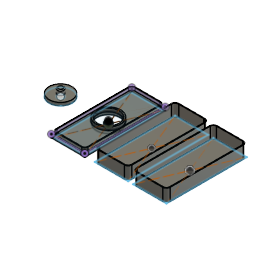
insert (Autodesk Fusion 360 design; units mm, degrees)
Autodesk Fusion 360 part; units mm, degrees
sketch "Sketch15" plane through (0, 0, 0) normal (0, 1, 0) x (1, 0, 0)
  line L0 (-335.7431, 132.5987) -> (-226.7431, 132.5987)
  line L1 (-226.7431, 132.5987) -> (-226.7431, -128.8013)
  line L2 (-226.7431, -128.8013) -> (-335.7431, -128.8013)
  line L3 (-335.7431, -128.8013) -> (-335.7431, 132.5987)
  line L4 (-335.7431, 132.5987) -> (-226.7431, -128.8013) construction
  line L5 (-226.7431, 132.5987) -> (-335.7431, -128.8013) construction
  line L6 (-228.7431, 130.5987) -> (-333.7431, 130.5987)
  line L7 (-333.7431, 130.5987) -> (-333.7431, -126.8013)
  line L8 (-333.7431, -126.8013) -> (-228.7431, -126.8013)
  line L9 (-228.7431, -126.8013) -> (-228.7431, 130.5987)
  line L10 (-228.7431, 130.5987) -> (-333.7431, -126.8013) construction
  line L11 (-333.7431, 130.5987) -> (-228.7431, -126.8013) construction
  point P0 (-281.2431, 1.8987)
  point P1 (-281.2431, 1.8987)
  dimension "d42" = 109
  dimension "d43" = 261.4
  dimension "d44" = 105
  dimension "d45" = 257.4
  constraint horizontal L0
  constraint perpendicular L0 L1
  constraint parallel L0 L2
  constraint parallel L1 L3
  constraint coincident L4 P1
  constraint coincident L5 P1
  constraint horizontal L6
  constraint perpendicular L6 L7
  constraint parallel L6 L8
  constraint parallel L7 L9
  constraint coincident L10 P1
  constraint coincident L11 P1
  constraint coincident P1 P0
  measures "d42" distance of L1.end L2.end
  measures "d43" distance of L0.end L1.end
  measures "d44" distance of L7.end L8.end
  measures "d45" distance of L6.end L7.end
extrude "Extrude9" add sketch "Sketch15" along normal blind 10 contours L6 L7 L8 L9 makes body 1
sketch "Sketch17" plane through (0, 0, 0) normal (0, 1, 0) x (1, 0, 0)
  line L0 (-210.9, 132.1) -> (-101.9, 132.1)
  line L1 (-101.9, 132.1) -> (-101.9, -129.3)
  line L2 (-101.9, -129.3) -> (-210.9, -129.3)
  line L3 (-210.9, -129.3) -> (-210.9, 132.1)
  line L4 (-210.9, 132.1) -> (-101.9, -129.3) construction
  line L5 (-101.9, 132.1) -> (-210.9, -129.3) construction
  line L6 (-103.9, 130.1) -> (-208.9, 130.1)
  line L7 (-208.9, 130.1) -> (-208.9, -127.3)
  line L8 (-208.9, -127.3) -> (-103.9, -127.3)
  line L9 (-103.9, -127.3) -> (-103.9, 130.1)
  line L10 (-103.9, 130.1) -> (-208.9, -127.3) construction
  point P0 (-156.4, 1.4)
  point P1 (-156.4, 1.4)
  dimension "d50" = 109
  dimension "d51" = 261.4
  dimension "d52" = 105
  dimension "d53" = 257.4
  constraint horizontal L0
  constraint perpendicular L0 L1
  constraint parallel L0 L2
  constraint parallel L1 L3
  constraint coincident L4 P1
  constraint coincident L5 P1
  constraint horizontal L6
  constraint perpendicular L6 L7
  constraint parallel L6 L8
  constraint parallel L7 L9
  constraint coincident L10 P1
  constraint coincident P1 P0
  measures "d50" distance of L1.end L2.end
  measures "d51" distance of L0.end L1.end
  measures "d52" distance of L7.end L8.end
  measures "d53" distance of L6.end L7.end
sketch "Sketch35" plane through (0, 0, 0) normal (0, 1, 0) x (1, 0, 0)
  line L0 (-365.7, 130.7) -> (-474.3, 130.7)
  line L1 (-474.3, 130.7) -> (-474.3, -130.7)
  line L2 (-474.3, -130.7) -> (-365.7, -130.7)
  line L3 (-365.7, -130.7) -> (-365.7, 130.7)
  line L4 (-365.7, 130.7) -> (-474.3, -130.7) construction
  line L5 (-474.3, 130.7) -> (-365.7, -130.7) construction
  circle A0 centre (-420, 0) radius 37.5
  point P0 (-420, 0)
  dimension "d73" = 108.6
  dimension "d82" = 75
  dimension "d111" = 261.4
  constraint horizontal L0
  constraint perpendicular L0 L1
  constraint parallel L0 L2
  constraint parallel L1 L3
  constraint coincident L4 P0
  constraint coincident L5 P0
  constraint coincident P0 A0.centre
  measures "d73" distance of L1.end L2.end
  measures "d82" diameter of A0
  measures "d111" distance of L0.end L1.end
sketch "Sketch37" plane through (0, 0, 0) normal (0, 1, 0) x (1, 0, 0)
  line L0 (-368.1512, 128.0997) -> (-471.8512, 128.0997)
  line L1 (-471.8512, 128.0997) -> (-471.8512, -128.1003)
  line L2 (-471.8512, -128.1003) -> (-368.1512, -128.1003)
  line L3 (-368.1512, -128.1003) -> (-368.1512, 128.0997)
  line L4 (-368.1512, 128.0997) -> (-471.8512, -128.1003) construction
  line L5 (-471.8512, 128.0997) -> (-368.1512, -128.1003) construction
  line L6 (-370.1512, 126.0997) -> (-469.8512, 126.0997)
  line L7 (-469.8512, 126.0997) -> (-469.8512, -126.1003)
  line L8 (-469.8512, -126.1003) -> (-370.1512, -126.1003)
  line L9 (-370.1512, -126.1003) -> (-370.1512, 126.0997)
  line L10 (-370.1512, 126.0997) -> (-469.8512, -126.1003) construction
  line L11 (-469.8512, 126.0997) -> (-370.1512, -126.1003) construction
  point P0 (-420.0012, -0.0003)
  point P1 (-420.0012, -0.0003)
  dimension "d76" = 103.7
  dimension "d77" = 256.2
  dimension "d78" = 99.7
  dimension "d79" = 252.2
  constraint horizontal L0
  constraint perpendicular L0 L1
  constraint parallel L0 L2
  constraint parallel L1 L3
  constraint coincident L4 P1
  constraint coincident L5 P1
  constraint horizontal L6
  constraint perpendicular L6 L7
  constraint parallel L6 L8
  constraint parallel L7 L9
  constraint coincident L10 P1
  constraint coincident L11 P1
  constraint coincident P1 P0
  measures "d76" distance of L1.end L2.end
  measures "d77" distance of L0.end L1.end
  measures "d78" distance of L7.end L8.end
  measures "d79" distance of L6.end L7.end
extrude "Extrude15" add sketch "Sketch35" along normal blind 10 makes body 2
sketch "Sketch42" plane through (0, 0, 0) normal (0, 1, 0) x (1, 0, 0)
sketch "Sketch45" plane through (0, 10, 0) normal (0, 1, 0) x (-1, 0, 0)
  circle A0 centre (420, 0) radius 37.5
  circle A1 centre (420, 0) radius 40
  circle A2 centre (420, 0) radius 35
  line L0 (365.7, 130.7) -> (365.7, -130.7)
  line L1 (365.7, -130.7) -> (474.3, -130.7)
  line L2 (474.3, -130.7) -> (474.3, 130.7)
  line L3 (474.3, 130.7) -> (365.7, 130.7)
  dimension "d91" = 80
  dimension "d92" = 70
  constraint concentric A0 A1
  constraint concentric A0 A2
  measures "d91" diameter of A1
  measures "d92" diameter of A2
extrude "Extrude18" add sketch "Sketch45" along normal blind 5 contours A0 | A1 bodies 2
sketch "Sketch48" plane through (0, 0, 0) normal (0, 1, 0) x (1, 0, 0)
  circle A0 centre (-575, 0) radius 37.2
  circle A1 centre (-575, 0) radius 10
  dimension "d95" = 74.4
  dimension "d96" = 20
  constraint concentric A0 A1
  measures "d95" diameter of A0
  measures "d96" diameter of A1
extrude "Extrude19" add sketch "Sketch48" along normal blind 25 separate body contours A1 makes body 3
extrude "Extrude20" add sketch "Sketch48" along normal blind 9.6 bodies 3
fillet "Fillet1" radius 3 1 edges at (-584.3233, 25, 3.6162) on bodies 3
extrude "Extrude28" cut 1 faces at (-263.7431, 10, -44.7987) along direction (0, -1, 0) blind 8 on bodies 1 bodies 1
extrude "Extrude30" cut 1 faces at (-420.9964, 10, 100.4294) along direction (0, -1, 0) blind 8 on bodies 2 bodies 2
extrude "Extrude31" add sketch "Sketch15" along normal blind 40 bodies 1
fillet "Fillet38" radius 10 1 edges at (-333.7431, 21, 126.8013) on bodies 1
fillet "Fillet39" radius 10 1 edges at (-228.7431, 21, 126.8013) on bodies 1
fillet "Fillet40" radius 10 1 edges at (-228.7431, 21, -130.5987) on bodies 1
fillet "Fillet41" radius 10 1 edges at (-333.7431, 21, -130.5987) on bodies 1
fillet "Fillet42" radius 10 1 edges at (-226.7431, 20, 128.8013) on bodies 1
fillet "Fillet43" radius 10 1 edges at (-335.7431, 20, 128.8013) on bodies 1
fillet "Fillet44" radius 10 1 edges at (-335.7431, 20, -132.5987) on bodies 1
fillet "Fillet45" radius 10 1 edges at (-226.7431, 20, -132.5987) on bodies 1
extrude "Extrude34" add sketch "Sketch35" along normal blind 10 separate body makes body 4
extrude "Extrude36" add sketch "Sketch45" along normal blind 10 contours A1 bodies 4
extrude "Extrude37" add sketch "Sketch45" along normal blind 10 contours A0 bodies 4
form "Form1" [no effect]
extrude "Extrude38" add sketch "Sketch37" along normal blind 20 separate body makes body 5
fillet "Fillet64" radius 8 1 edges at (-469.8512, 10, 126.1003) on bodies 5
fillet "Fillet65" radius 8 1 edges at (-469.8512, 10, -126.0997) on bodies 5
fillet "Fillet66" radius 8 1 edges at (-370.1512, 10, -126.0997) on bodies 5
fillet "Fillet67" radius 8 1 edges at (-370.1512, 10, 126.1003) on bodies 5
fillet "Fillet68" radius 10 1 edges at (-368.1512, 10, 128.1003) on bodies 5
fillet "Fillet69" radius 10 1 edges at (-471.8512, 10, 128.1003) on bodies 5
fillet "Fillet70" radius 10 1 edges at (-471.8512, 10, -128.0997) on bodies 5
fillet "Fillet71" radius 10 1 edges at (-474.3, 5, -130.7) on bodies 4
fillet "Fillet72" radius 10 1 edges at (-474.3, 5, 130.7) on bodies 4
fillet "Fillet73" radius 10 1 edges at (-365.7, 5, 130.7) on bodies 4
fillet "Fillet74" radius 10 1 edges at (-368.1512, 10, -128.0997) on bodies 5
fillet "Fillet75" radius 10 1 edges at (-365.7, 5, -130.7) on bodies 4
combine "Combine1" operation add target body 5 tool bodies 4
extrude "Extrude39" add sketch "Sketch17" along normal blind 40 separate body makes body 6
extrude "Extrude40" add sketch "Sketch17" along normal blind 2 contours L6 L7 L8 L9 bodies 6
fillet "Fillet76" radius 20 1 edges at (-208.9, 21, 127.3) on bodies 6
fillet "Fillet77" radius 20 1 edges at (-208.9, 21, -130.1) on bodies 6
fillet "Fillet78" radius 20 1 edges at (-103.9, 21, -130.1) on bodies 6
fillet "Fillet79" radius 20 1 edges at (-103.9, 21, 127.3) on bodies 6
fillet "Fillet80" radius 20 1 edges at (-210.9, 20, -132.1) on bodies 6
fillet "Fillet81" radius 20 1 edges at (-101.9, 20, -132.1) on bodies 6
fillet "Fillet82" radius 20 1 edges at (-101.9, 20, 129.3) on bodies 6
fillet "Fillet83" radius 20 1 edges at (-210.9, 20, 129.3) on bodies 6
delete_face "DeleteFace3" 1 faces at (-195.6152, 26.6667, 128.7362) on bodies 6
delete_face "DeleteFace4" 1 faces at (-106.1789, 13.3333, 121.6632) on bodies 6
delete_face "DeleteFace5" 1 faces at (-195.4414, 14.6667, 126.2) on bodies 6
delete_face "DeleteFace6" 1 faces at (-104.4638, 27.3333, 112.0152) on bodies 6
delete_face "DeleteFace7" 1 faces at (-103.3326, 13.3333, -119.5332) on bodies 6
delete_face "DeleteFace8" 1 faces at (-195.6152, 13.3333, -131.5362) on bodies 6
delete_face "DeleteFace9" 1 faces at (-234.8506, 13.3333, -132.418) on bodies 1
delete_face "DeleteFace10" 1 faces at (-327.6356, 13.3333, -132.418) on bodies 1
delete_face "DeleteFace11" 1 faces at (-327.4597, 14.6667, -129.8824) on bodies 1
delete_face "DeleteFace12" 1 faces at (-238.2673, 14.6667, -130.5874) on bodies 1
delete_face "DeleteFace13" 1 faces at (-109.4253, 14.6667, -123.9016) on bodies 6
delete_face "DeleteFace14" 1 faces at (-193.6152, 27.3333, -129.5362) on bodies 6
delete_face "DeleteFace15" 1 faces at (-234.3855, 13.3333, 128.5194) on bodies 1
delete_face "DeleteFace16" 1 faces at (-329.0138, 13.3333, 128.2513) on bodies 1
delete_face "DeleteFace17" 1 faces at (-236.8506, 14.6667, 126.6206) on bodies 1
delete_face "DeleteFace18" 1 faces at (-327.4597, 14.6667, 126.085) on bodies 1
fillet "Fillet84" radius 10 1 edges at (-103.9, 21, -130.1) on bodies 6
fillet "Fillet85" radius 10 1 edges at (-103.9, 21, 127.3) on bodies 6
fillet "Fillet86" radius 10 1 edges at (-208.9, 21, 127.3) on bodies 6
fillet "Fillet87" radius 10 1 edges at (-208.9, 21, -130.1) on bodies 6
fillet "Fillet88" radius 12 1 edges at (-101.9, 20, -132.1) on bodies 6
fillet "Fillet89" radius 12 1 edges at (-210.9, 20, -132.1) on bodies 6
fillet "Fillet90" radius 12 1 edges at (-101.9, 20, 129.3) on bodies 6
fillet "Fillet91" radius 12 1 edges at (-210.9, 20, 129.3) on bodies 6
fillet "Fillet92" radius 12 1 edges at (-228.7431, 21, 126.8013) on bodies 1
fillet "Fillet93" radius 12 1 edges at (-333.7431, 21, 126.8013) on bodies 1
fillet "Fillet94" radius 12 2 edges at (-333.7431, 21, -130.5987) (-228.7431, 21, -130.5987) on bodies 1
fillet "Fillet95" radius 12 4 edges at (-335.7431, 20, -132.5987) (-226.7431, 20, -132.5987) (-335.7431, 20, 128.8013) (-226.7431, 20, 128.8013) on bodies 1
delete_face "DeleteFace19" 1 faces at (-369.5184, 3.3333, 128.5605) on bodies 5
delete_face "DeleteFace20" 1 faces at (-375.7936, 16.6667, 127.8184) on bodies 5
delete_face "DeleteFace21" 1 faces at (-373.3424, 3.3333, -130.4181) on bodies 5
delete_face "DeleteFace22" 1 faces at (-377.6754, 13.3333, -128.0884) on bodies 5
delete_face "DeleteFace23" 1 faces at (-464.7758, 3.3333, -130.6887) on bodies 5
delete_face "DeleteFace24" 1 faces at (-464.2088, 16.6667, -127.8178) on bodies 5
delete_face "DeleteFace25" 1 faces at (-466.1925, 3.3333, 130.5193) on bodies 5
delete_face "DeleteFace26" 1 faces at (-462.327, 13.3333, 128.0889) on bodies 5
delete_face "DeleteFace27" 1 faces at (-372.3613, 16.6667, 123.6209) on bodies 5
delete_face "DeleteFace28" 1 faces at (-467.3718, 13.3333, 123.8901) on bodies 5
delete_face "DeleteFace29" 1 faces at (-468.3678, 13.3333, -122.7402) on bodies 5
delete_face "DeleteFace30" 1 faces at (-376.2651, 13.3333, -125.8742) on bodies 5
fillet "Fillet96" radius 12 4 edges at (-469.8512, 15, 126.1003) (-370.1512, 15, 126.1003) (-469.8512, 15, -126.0997) (-370.1512, 15, -126.0997) on bodies 5
delete_face "DeleteFace31" 1 faces at (-466.1322, 16.6667, -122.7845) on bodies 5
delete_face "DeleteFace32" 1 faces at (-372.3763, 16.6667, -121.0604) on bodies 5
delete_face "DeleteFace33" 1 faces at (-376.1512, 16.6667, 124.4926) on bodies 5
delete_face "DeleteFace34" 1 faces at (-468.5172, 13.3333, 119.599) on bodies 5
fillet "Fillet97" radius 10 4 edges at (-370.1512, 15, 126.1003) (-469.8512, 15, 126.1003) (-469.8512, 15, -126.0997) (-370.1512, 15, -126.0997) on bodies 5
fillet "Fillet98" radius 10 4 edges at (-368.1512, 15, -128.0997) (-471.8512, 15, -128.0997) (-471.8512, 15, 128.1003) (-368.1512, 15, 128.1003) on bodies 5
fillet "Fillet99" radius 12 1 edges at (-365.7, 5, 130.7) on bodies 5
fillet "Fillet100" radius 12 3 edges at (-474.3, 5, 130.7) (-474.3, 5, -130.7) (-365.7, 5, -130.7) on bodies 5
hidden bodies 2
equation "d76 = 104 mm - 0.3 mm"
equation "d77 = 257.4 mm - 1.2 mm"
equation "d78 = 100 mm - 0.3 mm"
equation "d79 = 253.4 mm - 1.2 mm"
